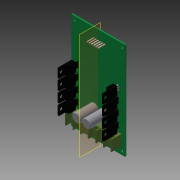
# Autodesk Inventor part: NyakMotorVezerlo
Saved by Autodesk Inventor 2015 (Build 190159000, 159)
## iProperties
Created: 2014-09-26
Part Number: NyakMotorVezerlo
Material: Generic
Document SubType Name: Modeling
Designer: laca
Density: 1 g/cm^3
Appearance: Default
Mass: 21.1726 g
Surface Area: 209.449 cm^2
Volume: 21.1726 cm^3
d0: 108.000 mm
d1: 60.000 mm
d2: 100.000 mm
d3: 53.000 mm
d4: 3.500 mm
d5: 4.000 mm
JukakANyakon: 3.000 mm
d7: 3.000 mm
d8: 3.000 mm
d9: 3.000 mm
d10: 1.500 mm
d11: 0.00 deg
d12: 1.500 mm
d13: 0.00 deg
d17: 8.000 mm
d18: 0.00 deg
d19: 10.000 mm
d20: 25.000 mm
d21: 1.100 mm
d22: 1.100 mm
d23: 0.200 mm
d26: 6.000 ul
d28: 2.450 mm
d29: 42.000 mm
d30: 8.000 mm
d31: 1.500 mm
d32: 1.000 mm
d33: 1.500 mm
d34: 1.000 mm
d35: 1.500 mm
d36: 1.000 mm
d37: 0.667 mm
d38: 0.667 mm
d40: 4.000 mm
d41: 0.00 deg
d42: 10.000 mm
d43: 5.000 mm
d44: 2.083 mm
d45: 1.500 mm
d47: 9.000 mm
d48: 0.00 deg
d49: 1.500 mm
d50: 6.500 mm
d51: 0.00 deg
d52: 3.500 mm
d54: 25.00 deg
d55: 4.000 ul
d57: 12.000 mm
TranzisztoJukAtmero: 4.000 mm
d59: 5.000 mm
d60: 3.000 mm
d62: 0.00 deg
d63: 12.000 mm
d64: 52.000 mm
d65: 4.000 mm
d66: 8.000 mm
d69: 6.000 mm
d70: 0.00 deg
d71: 1.000 mm
d72: 5.000 mm
d73: 0.00 deg
d74: 7.000 ul
d76: 8.497 mm
d77: 10.000 mm
d78: 10.000 mm
d79: 0.000 mm
d80: 11.000 mm
d81: 30.000 mm
d82: 20.000 mm
d83: 0.00 deg
d84: 1.000 mm
JukakKoztiTavolsagSzeleseg: 53.000 mm
JukaKoztiTavolsagHoszusag: 100.000 mm
Author: laca
Autodesk Inventor part; units mm, degrees
ref_plane "YZ Plane" through (0, 0, 0) normal (1, 0, 0) x (0, 1, 0)
ref_plane "XZ Plane" through (0, 0, 0) normal (0, 1, 0) x (-1, 0, 0)
ref_plane "XY Plane" through (0, 0, 0) normal (0, 0, 1) x (1, 0, 0)
sketch "Sketch1" plane through (0, 0, 0) normal (0, 1, 0) x (-1, 0, 0)
  line L0 (8.506, 15.8805) -> (-51.494, 15.8805)
  line L1 (-51.494, 15.8805) -> (-51.494, -92.1195)
  line L2 (-51.494, -92.1195) -> (8.506, -92.1195)
  line L3 (8.506, -92.1195) -> (8.506, 15.8805)
  line L4 (-47.994, 11.8805) -> (5.006, 11.8805)
  line L5 (5.006, 11.8805) -> (5.006, -88.1195)
  line L6 (5.006, -88.1195) -> (-47.994, -88.1195)
  line L7 (-47.994, -88.1195) -> (-47.994, 11.8805)
  circle A0 centre (5.006, 11.8805) radius 1.5
  circle A1 centre (5.006, -88.1195) radius 1.5
  circle A2 centre (-47.994, -88.1195) radius 1.5
  circle A3 centre (-47.994, 11.8805) radius 1.5
  point P0 (0, 0)
  dimension "d0" = 108
  dimension "d1" = 60
  dimension "JukaKoztiTavolsagHoszusag" = 100
  dimension "JukakKoztiTavolsagSzeleseg" = 53
  dimension "d4" = 3.5
  dimension "d5" = 4
  dimension "JukakANyakon" = 3
  dimension "d7" = 3
  dimension "d8" = 3
  dimension "d9" = 3
  constraints: 16 end point, 4 centre point, 4 coincident, 4 parallel, 2 horizontal, 2 perpendicular
  measures "d0" distance of L2.end L0.start
  measures "d1" distance of L0.start L0.end
  measures "JukaKoztiTavolsagHoszusag" distance of L4.end L5.end
  measures "JukakKoztiTavolsagSzeleseg" distance of L4.start L4.end
  measures "d4" distance between parallel lines of L3 L5
  measures "d5" distance between parallel lines of L0 L4
  measures "JukakANyakon" diameter of A0
  measures "d7" diameter of A1
  measures "d8" diameter of A2
  measures "d9" diameter of A3
extrude "Extrusion1" add sketch "Sketch1" along normal blind 1.5 contours L3 L2 L1 L0 | L4 A3 L7 | L4 A0 L5 A1 L6 A2 L7 A3 | L4 L5 A0 | A2 L6 L7 | L5 L6 A1 picked at (-47.6658, 10.9426) picked at (4.8947, 10.893) picked at (-47.2913, -87.4168) picked at (4.1646, -87.5908)
extrude "Extrusion2" cut sketch "Sketch1" along normal blind 1.5 contours L7 A3 L4 | L4 A3 L7 | A0 L5 L4 | L4 L5 A0 | A2 L6 L7 | L7 L6 A2 | A1 L6 L5 | L5 L6 A1
sketch "Sketch2" plane through (0, 0, 0) normal (0, -1, 0) x (1, 0, 0)
  line L0 (-8.506, 15.8805) -> (51.494, 15.8805) projected
  line L1 (-8.506, -92.1195) -> (-8.506, 15.8805) projected
  line L2 (16.494, 5.8805) -> (17.594, 5.8805)
  line L3 (17.594, 5.8805) -> (17.594, 4.7805)
  line L4 (17.594, 4.7805) -> (16.494, 4.7805)
  line L5 (16.494, 4.7805) -> (16.494, 5.8805)
  line L6 (44.494, -26.1195) -> (43.494, -26.1195)
  line L7 (43.494, -26.1195) -> (43.494, -27.6195)
  line L8 (43.494, -27.6195) -> (44.494, -27.6195)
  line L9 (44.494, -27.6195) -> (44.494, -26.1195)
  line L10 (51.494, 15.8805) -> (51.494, -92.1195) projected
  line L11 (44.494, -28.2862) -> (43.494, -28.2862)
  line L12 (43.494, -28.2862) -> (43.494, -29.7862)
  line L13 (43.494, -29.7862) -> (44.494, -29.7862)
  line L14 (44.494, -29.7862) -> (44.494, -28.2862)
  line L15 (44.494, -30.4528) -> (43.494, -30.4528)
  line L16 (43.494, -30.4528) -> (43.494, -31.9528)
  line L17 (43.494, -31.9528) -> (44.494, -31.9528)
  line L18 (44.494, -31.9528) -> (44.494, -30.4528)
  point P0 (0, 0)
  dimension "d19" = 10
  dimension "d20" = 25
  dimension "d21" = 1.1
  dimension "d22" = 1.1
  dimension "d29" = 42
  dimension "d30" = 8
  dimension "d31" = 1.5
  dimension "d32" = 1
  dimension "d33" = 1.5
  dimension "d34" = 1
  dimension "d35" = 1.5
  dimension "d36" = 1
  dimension "d37" = 0.6667
  dimension "d38" = 0.6667
  dimension "d39" = 5.8333
  constraints: 32 end point, 8 parallel, 4 horizontal, 4 perpendicular, 2 collinear
  measures "d19" distance between parallel lines of L0 L2
  measures "d20" distance between parallel lines of L1 L5
  measures "d21" distance of L3.end L4.end
  measures "d22" distance of L2.end L3.end
  measures "d29" distance between parallel lines of L0 L6
  measures "d30" distance between parallel lines of L10 L7
  measures "d31" distance of L6.end L7.end
  measures "d32" distance of L7.end L8.end
  measures "d33" distance of L11.end L12.end
  measures "d34" distance of L12.end L13.end
  measures "d35" distance of L15.end L16.end
  measures "d36" distance of L16.end L17.end
  measures "d37" distance from line of L11 L7.end
  measures "d38" distance between parallel lines of L15 L13
  measures "d39" distance between parallel lines of L17 L6
extrude "Extrusion3" add sketch "Sketch2" along normal blind 8 contours L2 L3 L4 L5
chamfer "Chamfer1" distance 0.2 angle 45 4 edges at (17.594, -8, 5.3305) (17.044, -8, 5.8805) (16.494, -8, 5.3305) (17.044, -8, 4.7805)
pattern_linear "Rectangular Pattern1" count 6 spacing 2.45 along (1, 0, 0) of "Extrusion3", "Chamfer1"
extrude "Extrusion4" add sketch "Sketch2" along normal blind 4 contours L9 L8 L7 L6 | L14 L13 L12 L11 | L18 L17 L16 L15
sketch "Sketch3" plane through (0, -4, 0) normal (0, -1, 0) x (1, 0, 0)
  line L0 (41.994, -24.0362) -> (46.994, -24.0362)
  line L1 (46.994, -24.0362) -> (46.994, -34.0362)
  line L2 (46.994, -34.0362) -> (41.994, -34.0362)
  line L3 (41.994, -34.0362) -> (41.994, -24.0362)
  line L4 (44.494, -26.1195) -> (43.494, -26.1195) projected
  line L5 (43.494, -26.1195) -> (43.494, -27.6195) projected
  line L6 (43.494, -31.9528) -> (44.494, -31.9528) projected
  point P0 (0, 0)
  dimension "d42" = 10
  dimension "d43" = 5
  dimension "d44" = 2.0833
  dimension "d45" = 1.5
  dimension "d46" = 5.8333
  constraints: 8 end point, 2 parallel, 1 horizontal, 1 perpendicular
  measures "d42" distance of L2.end L0.start
  measures "d43" distance of L0.start L0.end
  measures "d44" distance between parallel lines of L0 L4
  measures "d45" distance between parallel lines of L3 L5
  measures "d46" distance between parallel lines of L4 L6
extrude "Extrusion5" add sketch "Sketch3" along normal blind 9
sketch "Sketch4" plane through (0, -13, 0) normal (0, -1, 0) x (1, 0, 0)
  line L0 (41.994, -34.0362) -> (46.994, -34.0362) projected
  line L1 (46.994, -24.0362) -> (45.494, -24.0362)
  line L2 (45.494, -24.0362) -> (45.494, -34.0362)
  line L3 (45.494, -34.0362) -> (46.994, -34.0362)
  line L4 (46.994, -34.0362) -> (46.994, -24.0362)
  point P0 (0, 0)
  dimension "d49" = 1.5
  constraints: 8 end point, 2 parallel, 1 horizontal, 1 perpendicular, 1 point on line
  measures "d49" distance of L1.start L1.end
extrude "Extrusion6" add sketch "Sketch4" along normal blind 6.5
chamfer "Chamfer2" distance 3.5 angle 25 1 edges at (41.994, -13, -29.0362) measured on face at (43.1607, -13, -30.7028)
sketch "Sketch5" plane through (45.494, -19.5, -34.0362) normal (-1, 0, 0) x (0, 0, 1)
  circle A0 centre (5, 3) radius 2
  line L0 (10, 6.5) -> (10, 0) projected
  line L1 (10, 0) -> (0, 0) projected
  point P0 (34.0362, 19.5)
  dimension "TranzisztoJukAtmero" = 4
  dimension "d59" = 5
  dimension "d60" = 3
  constraints: 1 centre point
  measures "TranzisztoJukAtmero" diameter of A0
  measures "d59" distance from line of L0 A0.centre
  measures "d60" distance from line of A0.centre L1
extrude "Extrusion7" cut sketch "Sketch5" against normal through all
pattern_linear "Rectangular Pattern2" count 4 spacing 12 along (0, 0, -1) of "Extrusion4", "Extrusion5", "Extrusion6", "Chamfer2", "Extrusion7"
ref_plane "Work Plane1" through (21.494, 0, 15.8805) normal (1, 0, 0) x (0, 0, -1)
mirror "Mirror1" about plane through (21.494, 0, 15.8805) normal (1, 0, 0) of "Extrusion4", "Extrusion5", "Extrusion6", "Chamfer2", "Extrusion7", "Rectangular Pattern2"
sketch "Sketch6" plane through (0, 0, 0) normal (0, -1, 0) x (1, 0, 0)
  line L0 (-4.506, -72.1195) -> (47.494, -72.1195)
  line L1 (47.494, -72.1195) -> (47.494, -84.1195)
  line L2 (47.494, -84.1195) -> (-4.506, -84.1195)
  line L3 (-4.506, -84.1195) -> (-4.506, -72.1195)
  line L4 (-8.506, -92.1195) -> (-8.506, 15.8805) projected
  line L5 (51.494, -92.1195) -> (-8.506, -92.1195) projected
  line L6 (41.994, -70.0362) -> (45.494, -70.0362) projected
  line L7 (46.994, -24.0362) -> (45.494, -24.0362) projected
  point P0 (0, 0)
  dimension "d63" = 12
  dimension "d64" = 52
  dimension "d65" = 4
  dimension "d66" = 8
  dimension "d67" = 60
  dimension "d68" = 46
  constraints: 8 end point, 2 parallel, 1 horizontal, 1 perpendicular
  measures "d63" distance of L2.end L0.start
  measures "d64" distance of L0.start L0.end
  measures "d65" distance between parallel lines of L4 L3
  measures "d66" distance between parallel lines of L5 L2
  measures "d67" distance of L5.start L4.start
  measures "d68" distance between parallel lines of L6 L7
extrude "Extrusion8" add sketch "Sketch6" along normal blind 6
sketch "Sketch7" plane through (0, -6, 0) normal (0, -1, 0) x (1, 0, 0)
  line L0 (-4.506, -84.1195) -> (47.494, -84.1195) projected
  line L1 (-4.506, -72.1195) -> (-3.506, -72.1195)
  line L2 (-3.506, -72.1195) -> (-3.506, -84.1195)
  line L3 (-3.506, -84.1195) -> (-4.506, -84.1195)
  line L4 (-4.506, -84.1195) -> (-4.506, -72.1195)
  point P0 (0, 0)
  dimension "d71" = 1
  constraints: 8 end point, 2 parallel, 1 horizontal, 1 perpendicular, 1 point on line
  measures "d71" distance between parallel lines of L2 L4
extrude "Extrusion9" add sketch "Sketch7" along normal blind 5
pattern_linear "Rectangular Pattern3" count 7 spacing 8.4967 along (1, 0, 0) of "Extrusion9"
sketch "Sketch8" plane through (0, 0, 0) normal (0, -1, 0) x (1, 0, 0)
  circle A0 centre (28.1768, -62.1195) radius 5
  circle A1 centre (17.1768, -62.1195) radius 5
  line L0 (51.494, -92.1195) -> (-8.506, -92.1195) projected
  point P0 (0, 0)
  dimension "d77" = 10
  dimension "d78" = 10
  dimension "d79" = 0
  dimension "d80" = 11
  dimension "d81" = 30
  constraints: 2 centre point
  measures "d77" diameter of A0
  measures "d78" diameter of A1
  measures "d79" vertical distance of A1.centre A0.centre
  measures "d80" distance of A1.centre A0.centre
  measures "d81" distance from line of L0 A0.centre
extrude "Extrusion10" add sketch "Sketch8" along normal blind 20
fillet "Fillet1" radius 1 2 edges at (12.1768, -20, -62.1195) (23.1768, -20, -62.1195)
equation "\"d4\" = -0.5 * JukakKoztiTavolsagSzeleseg + 0.5 * d1"
equation "\"d5\" = -0.5 * JukaKoztiTavolsagHoszusag + 0.5 * d0"
equation "\"d37\" = d38"
equation "\"d44\" = -0.5 * d46 + 0.5 * d42"
equation "\"d65\" = -0.5 * d64 + 0.5 * d67"
body "Solid1"
